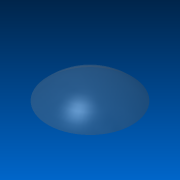
# Autodesk Inventor part: GoPro Hero 3 Lens
Saved by Autodesk Inventor 2015 (Build 190159000, 159)
## iProperties
Created: 2013-02-15
Material: Glass
Document SubType Name: Modeling
Designer: sdarley
Density: 1 g/cm^3
Project: GoPro Hero 3 HD Camera
Description: GoPro Hero 3 Lens
Appearance: Clear Reflective
Author: sdarley
Title: GoPro Hero 3 Lens
Revision Number: 1
Autodesk Inventor part; units mm, degrees
ref_plane "YZ Plane" through (0, 0, 0) normal (1, 0, 0) x (0, 1, 0)
ref_plane "XZ Plane" through (0, 0, 0) normal (0, 1, 0) x (-1, 0, 0)
ref_plane "XY Plane" through (0, 0, 0) normal (0, 0, 1) x (1, 0, 0)
sketch "Sketch1" plane through (0, 0, 0) normal (0, 1, 0) x (-1, 0, 0)
  line L0 (0, 2.9) -> (0, 3)
  line L1 (6.664, 0) -> (6.8, 0)
  arc A0 (6.664, 0) -> (0, 2.9) centre (0, -6.2067) ccw
  arc A1 (6.8, 0) -> (0, 3) centre (0, -6.2067) ccw
  point P0 (0, 0)
  dimension "d0" = 0.1
  dimension "d2" = 6.8
  dimension "d4" = 3
  constraints: 4 end point, 4 point on circle, 2 centre point, 1 concentric, 1 horizontal alignment, 1 line through centre, 1 perpendicular, 1 vertical, 1 vertical alignment
  measures "d0" radial gap between concentric circles of A0 A1
  measures "d2" distance of L1.end point (0, 0)
  measures "d4" distance of L0.end point (0, 0)
revolve "Revolution1" add sketch "Sketch1" angle 360 about axis through (0, 0, 2.9) along (0, 0, 1)
body "Solid1"
